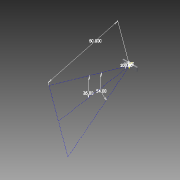
# Autodesk Inventor part: camera mount v1
Saved by Autodesk Inventor 2016 SP2 (Build 200236200, 236)
## iProperties
Created: 2016-09-20
Part Number: camera mount v1
Material: Generic
Document SubType Name: Modeling
Designer: hwasserb
Density: 1 g/cm^3
Appearance: Default
Author: hwasserb
Autodesk Inventor part; units mm, degrees
ref_plane "YZ Plane" through (0, 0, 0) normal (1, 0, 0) x (0, 1, 0)
ref_plane "XZ Plane" through (0, 0, 0) normal (0, 1, 0) x (-1, 0, 0)
ref_plane "XY Plane" through (0, 0, 0) normal (0, 0, 1) x (1, 0, 0)
sketch "Sketch1" plane through (0, 0, 0) normal (0, 0, 1) x (1, 0, 0)
  line L0 (0, 0) -> (304.8, 0)
  line L1 (304.8, 0) -> (304.8, -76.2)
  line L2 (304.8, -76.2) -> (0, -76.2)
  line L3 (0, -76.2) -> (0, 0)
  point P0 (0, 0)
  dimension "d0" = 304.8
  dimension "d1" = 76.2
  constraints: 8 end point, 2 parallel, 1 coincident, 1 horizontal, 1 perpendicular
  measures "d0" distance of L0.start L0.end
  measures "d1" distance of L2.end L0.start
extrude "Extrusion1" add sketch "Sketch1" along normal blind 25.4
sketch "Sketch2" plane through (0, 0, 0) normal (0, 0, -1) x (-1, 0, 0)
  line L0 (0, 0) -> (-304.8, 0) projected
  line L1 (0, -76.2) -> (0, 0) projected
  line L2 (-228.6, -25.4) -> (-203.2, -25.4)
  line L3 (-203.2, -25.4) -> (-203.2, -31.75)
  line L4 (-203.2, -31.75) -> (-228.6, -31.75)
  line L5 (-228.6, -31.75) -> (-228.6, -25.4)
  line L6 (-101.6, -25.4) -> (-76.2, -25.4)
  line L7 (-76.2, -25.4) -> (-76.2, -31.75)
  line L8 (-76.2, -31.75) -> (-101.6, -31.75)
  line L9 (-101.6, -31.75) -> (-101.6, -25.4)
  dimension "d4" = 25.4
  dimension "d5" = 6.35
  dimension "d6" = 101.6
  dimension "d7" = 76.2
  dimension "d9" = 25.4
  constraints: 16 end point, 4 parallel, 2 equal length, 2 horizontal, 2 perpendicular, 1 collinear
  measures "d4" distance of L2.start L2.end
  measures "d5" distance of L4.end L2.start
  measures "d6" distance between parallel lines of L9 L3
  measures "d7" distance between parallel lines of L1 L7
  measures "d9" distance between parallel lines of L6 L0
extrude "Extrusion2" add sketch "Sketch2" along normal blind 25.4
sketch "Sketch3" plane through (76.2, -25.4, 0) normal (0, 1, 0) x (1, 0, 0)
  line L0 (0, 25.4) -> (25.4, 25.4) projected
  line L1 (0, 0) -> (0, 25.4) projected
  line L2 (127, 0) -> (127, 25.4) projected
  point P0 (-76.2, 0)
  point P1 (12.7, 12.7)
  point P2 (139.7, 12.7)
  dimension "d12" = 12.7
  dimension "d13" = 12.7
  dimension "d14" = 12.7
  constraints: 1 horizontal alignment
  measures "d12" distance from line of point (12.7, 12.7) L1
  measures "d13" distance from line of L2 point (139.7, 12.7)
  measures "d14" distance from line of L0 point (12.7, 12.7)
hole "Hole1" at (88.9, -25.4, -12.7) at (215.9, -25.4, -12.7) direction (0, -1, 0) diameter 6.35 end through all
ref_plane "Work Plane1" through (152.4, -76.2, 0) normal (1, 0, 0) x (0, 0, -1)
sketch "Sketch4" plane through (152.4, -76.2, 0) normal (1, 0, 0) x (0, 0, -1)
  line L0 (-25.4, 0) -> (-25.4, 76.2) projected
  line L1 (-25.4, 38.1) -> (-1731.7329, 527.3831) construction
  line L2 (-1731.7329, 527.3831) -> (-1331.5316, -982.3618) construction
  line L3 (-1331.5316, -982.3618) -> (-25.4, 38.1) construction
  line L4 (-25.4, 38.1) -> (-1531.6322, -227.4894) construction
  point P0 (0, 76.2)
  dimension "d26" = 54
  dimension "d27" = 38.1
  dimension "d28" = 26
  dimension "d29" = 1524
  dimension "d30" = 100
  constraints: 8 end point, 2 midpoint
  measures "d26" angle of L1 L3
  measures "d27" distance of L0.end L1.start
  measures "d28" angle of L1 L4
  measures "d29" distance from line of L2 L1.start
  measures "d30" angle of L0 L4
body "Solid1"
